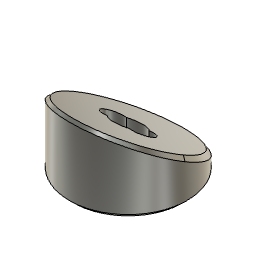
Screen Door Spacer v2 (Autodesk Fusion 360 design; units mm, degrees)
Autodesk Fusion 360 part; units mm, degrees
sketch "Sketch1" plane through (0, 0, 0) normal (0, 1, 0) x (1, 0, 0)
  line L0 (0, 0) -> (16, 0)
  line L1 (16, 0) -> (16, -20.5)
  line L2 (16, -20.5) -> (0, -20.5)
  line L3 (0, -20.5) -> (0, 0)
  dimension "d1" = 16
  dimension "d2" = 20.5
  constraint horizontal L0
  constraint vertical L1
  constraint horizontal L2
  constraint vertical L3
  constraint coincident L0.start L3.end
  measures "d1" distance of L0.start L0.end
  measures "d2" distance of L0.start L2.end
revolve "Revolve1" add sketch "Sketch1" angle 360 about axis through (0, 0, 1.75) along (0, 0, 1)
sketch "Sketch2" plane through (0, 0, 0) normal (0, 0, 1) x (1, 0, 0)
  circle A0 centre (0, 0) radius 4
  circle A1 centre (-4, 0) radius 2.75
  circle A2 centre (4, 0) radius 2.75
  dimension "d4" = 8
  dimension "d5" = 5.5
  dimension "d6" = 5.5
  constraint coincident A0.centre origin
  constraint coincident A0 A1.centre
  constraint coincident A0 A2.centre
  measures "d4" diameter of A0
  measures "d5" diameter of A1
  measures "d6" diameter of A2
extrude "Extrude1" cut sketch "Sketch2" along normal blind 18
sketch "Sketch4" plane through (0, 0, 0) normal (1, 0, 0) x (0, 1, 0)
  line L0 (-16, 20.5) -> (17.4115, 1.2099)
  line L1 (-16, 20.5) -> (22.5802, 20.5) construction
  line L2 (17.4115, 1.2099) -> (17.4115, 23.2935)
  line L3 (17.4115, 23.2935) -> (-18.7397, 23.2935)
  line L4 (-18.7397, 23.2935) -> (-16, 20.5)
  dimension "d9" = 30
  constraint horizontal L1
  constraint perpendicular L1 L2
  constraint perpendicular L2 L3
  measures "d9" angle of L0 L1
extrude "Extrude2" cut sketch "Sketch4" along normal blind 16 and the other way blind 16
chamfer "Chamfer1" distance 1 angle 45 2 edges at (0, -16, 20.5) (-14.9172, -5.7858, 0)
